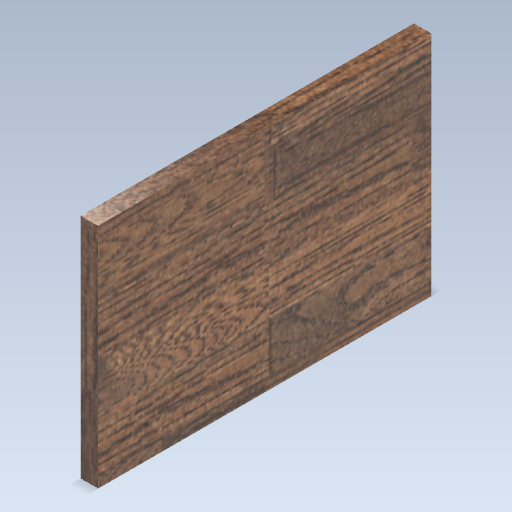
# Autodesk Inventor part: Control Box Cover
Saved by Autodesk Inventor 2020 (Build 240168000, 168)
## iProperties
Created: 2020-08-16
Part Number: Control Box Cover
Material: Generic
Document SubType Name: Modeling
Designer: Abbas
Density: 1 g/cm^3
Appearance: Default
Author: Abbas
Autodesk Inventor part; units mm, degrees
ref_plane "YZ Plane" through (0, 0, 0) normal (1, 0, 0) x (0, 1, 0)
ref_plane "XZ Plane" through (0, 0, 0) normal (0, 1, 0) x (-1, 0, 0)
ref_plane "XY Plane" through (0, 0, 0) normal (0, 0, 1) x (1, 0, 0)
sketch "Sketch1" plane through (0, 0, 0) normal (1, 0, 0) x (0, 1, 0)
  line L0 (-130, 188.914) -> (-130, -192)
  line L1 (-130, -192) -> (130, -192)
  line L2 (130, -192) -> (130, 188.914)
  line L3 (130, 188.914) -> (-130, 188.914)
  line L4 (130, 188.914) -> (390, 188.914) construction
  dimension "d0" = 260
  dimension "d15" = 180
  constraints: 10 end point, 1 collinear, 1 horizontal, 1 parallel
  measures "d0" distance of L1.end L0.end
  measures "d15" angle of L3 L4
extrude "Extrusion1" add sketch "Sketch1" along normal blind 20
sketch "Sketch2" plane through (0, -130, -192) normal (0, 0, -1) x (-1, 0, 0)
  circle A0 centre (-13, 244.99) radius 1.875
  circle A1 centre (-13, 219.19) radius 1.875
  circle A2 centre (-13, 193.39) radius 1.875
  line L0 (0, 260) -> (-20, 260) projected
  line L1 (0, 0) -> (0, 260) projected
  point P0 (0, 130)
  dimension "d4" = 3.75
  dimension "d5" = 3.75
  dimension "d6" = 3.75
  dimension "d7" = 15.01
  dimension "d8" = 25.8
  dimension "d9" = 25.8
  dimension "d10" = 13
  constraints: 3 centre point
  measures "d4" diameter of A0
  measures "d5" diameter of A1
  measures "d6" diameter of A2
  measures "d7" distance from line of L0 A0.centre
  measures "d8" distance of A0.centre A1.centre
  measures "d9" distance of A1.centre A2.centre
  measures "d10" distance from line of L1 A0.centre
extrude "Extrusion2" cut sketch "Sketch2" against normal blind 10
body "Solid1"
